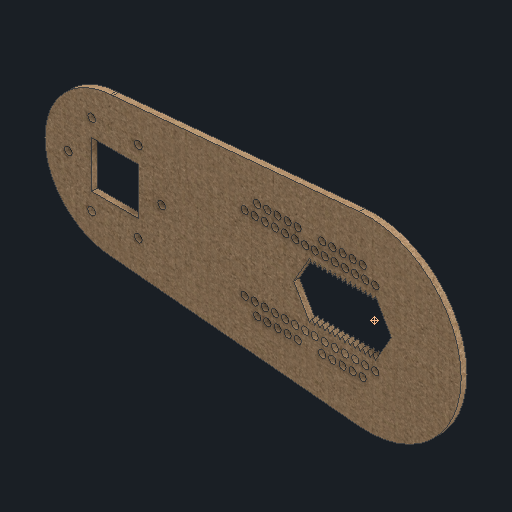
# Autodesk Inventor part: WeightArm
Saved by Autodesk Inventor 2024.1 (Build 281209000, 209)
## iProperties
Created: 2023-10-16
Part Number: WeightArm
Material: MDF Medium Density Fiberboard
Document SubType Name: Modeling
Designer: Brandon
Density: 0.8 g/cm^3
Appearance: Cardboard - Corrugated
Mass: 33.1484 g
Surface Area: 289.834 cm^2
Volume: 41.4355 cm^3
Author: Brandon
Autodesk Inventor part; units mm, degrees
ref_plane "YZ Plane" through (0, 0, 0) normal (1, 0, 0) x (0, 1, 0)
ref_plane "XZ Plane" through (0, 0, 0) normal (0, 1, 0) x (-1, 0, 0)
ref_plane "XY Plane" through (0, 0, 0) normal (0, 0, 1) x (1, 0, 0)
sketch "Sketch1" plane through (0, 0, 0) normal (0, 0, 1) x (1, 0, 0)
  line L0 (-285.1848, -19.0386) -> (264.1554, -38.0771) projected
  arc A0 (264.1554, -38.0771) -> (264.1554, 38.0771) centre (265.475, 0) ccw projected
  line L1 (264.1554, 38.0771) -> (-285.1848, 19.0386) projected
  arc A1 (-285.1848, 19.0386) -> (-285.1848, -19.0386) centre (-284.525, 0) ccw projected
  circle A2 centre (-284.525, -9.525) radius 2 projected
  circle A3 centre (-294.05, 0) radius 2 projected
  circle A4 centre (-284.525, 9.525) radius 2 projected
  circle A5 centre (290.875, 0) radius 2.1 projected
  circle A6 centre (278.175, -21.997) radius 2.1 projected
  circle A7 centre (252.775, -21.997) radius 2.1 projected
  circle A8 centre (278.175, 21.997) radius 2.1 projected
  circle A9 centre (252.775, 21.997) radius 2.1 projected
  line L2 (252.775, -12.7) -> (252.775, 12.7) projected
  line L3 (252.775, 12.7) -> (278.175, 12.7) projected
  line L4 (278.175, 12.7) -> (278.175, -12.7) projected
  line L5 (278.175, -12.7) -> (252.775, -12.7) projected
  circle A10 centre (240.075, 0) radius 2.1 projected
  circle A11 centre (-275, 0) radius 2 projected
  circle A12 centre (265.475, 0) radius 38.1
  line L6 (265.475, 0) -> (402.975, 0)
  arc A13 (398.2829, -50.5828) -> (398.2829, 50.5828) centre (402.975, 0) ccw
  line L7 (261.9559, 37.9371) -> (398.2829, 50.5828)
  line L8 (265.475, 0) -> (375.475, 0)
  line L9 (402.975, 12.7) -> (402.975, -12.7)
  line L10 (404.35, 12.7) -> (401.6, 12.7)
  line L11 (402.975, 12.7) -> (404.35, 15.0816)
  line L12 (402.975, 12.7) -> (405.725, 12.7) construction
  line L13 (404.35, 15.0816) -> (405.725, 12.7)
  line L14 (405.725, 12.7) -> (407.1, 15.0816)
  line L15 (405.725, 12.7) -> (408.475, 12.7) construction
  line L16 (407.1, 15.0816) -> (408.475, 12.7)
  line L17 (402.975, -12.7) -> (404.35, -15.0816)
  line L18 (402.975, -12.7) -> (405.725, -12.7) construction
  line L19 (404.35, -15.0816) -> (405.725, -12.7)
  line L20 (405.725, -12.7) -> (407.1, -15.0816)
  line L21 (405.725, -12.7) -> (408.475, -12.7) construction
  line L22 (407.1, -15.0816) -> (408.475, -12.7)
  line L23 (397.475, 12.7) -> (398.85, 15.0816)
  line L24 (398.85, 15.0816) -> (400.225, 12.7)
  line L25 (397.475, 12.7) -> (400.225, 12.7) construction
  line L26 (400.225, 12.7) -> (401.6, 15.0816)
  line L27 (401.6, 15.0816) -> (402.975, 12.7)
  line L28 (400.225, 12.7) -> (402.975, 12.7) construction
  line L29 (397.475, -12.7) -> (398.85, -15.0816)
  line L30 (397.475, -12.7) -> (400.225, -12.7) construction
  line L31 (400.225, -12.7) -> (401.6, -15.0816)
  line L32 (400.225, -12.7) -> (402.975, -12.7) construction
  line L33 (401.6, -15.0816) -> (402.975, -12.7)
  line L34 (398.85, -15.0816) -> (400.225, -12.7)
  line L35 (391.975, 12.7) -> (393.35, 15.0816)
  line L36 (393.35, 15.0816) -> (394.725, 12.7)
  line L37 (391.975, 12.7) -> (394.725, 12.7) construction
  line L38 (394.725, 12.7) -> (396.1, 15.0816)
  line L39 (396.1, 15.0816) -> (397.475, 12.7)
  line L40 (394.725, 12.7) -> (397.475, 12.7) construction
  line L41 (391.975, -12.7) -> (393.35, -15.0816)
  line L42 (391.975, -12.7) -> (394.725, -12.7) construction
  line L43 (394.725, -12.7) -> (396.1, -15.0816)
  line L44 (394.725, -12.7) -> (397.475, -12.7) construction
  line L45 (396.1, -15.0816) -> (397.475, -12.7)
  line L46 (393.35, -15.0816) -> (394.725, -12.7)
  line L47 (386.475, 12.7) -> (387.85, 15.0816)
  line L48 (387.85, 15.0816) -> (389.225, 12.7)
  line L49 (386.475, 12.7) -> (389.225, 12.7) construction
  line L50 (389.225, 12.7) -> (390.6, 15.0816)
  line L51 (390.6, 15.0816) -> (391.975, 12.7)
  line L52 (389.225, 12.7) -> (391.975, 12.7) construction
  line L53 (386.475, -12.7) -> (387.85, -15.0816)
  line L54 (386.475, -12.7) -> (389.225, -12.7) construction
  line L55 (389.225, -12.7) -> (390.6, -15.0816)
  line L56 (389.225, -12.7) -> (391.975, -12.7) construction
  line L57 (390.6, -15.0816) -> (391.975, -12.7)
  line L58 (387.85, -15.0816) -> (389.225, -12.7)
  line L59 (380.975, 12.7) -> (382.35, 15.0816)
  line L60 (382.35, 15.0816) -> (383.725, 12.7)
  line L61 (380.975, 12.7) -> (383.725, 12.7) construction
  line L62 (383.725, 12.7) -> (385.1, 15.0816)
  line L63 (385.1, 15.0816) -> (386.475, 12.7)
  line L64 (383.725, 12.7) -> (386.475, 12.7) construction
  line L65 (380.975, -12.7) -> (382.35, -15.0816)
  line L66 (380.975, -12.7) -> (383.725, -12.7) construction
  line L67 (383.725, -12.7) -> (385.1, -15.0816)
  line L68 (383.725, -12.7) -> (386.475, -12.7) construction
  line L69 (385.1, -15.0816) -> (386.475, -12.7)
  line L70 (382.35, -15.0816) -> (383.725, -12.7)
  line L71 (375.475, 12.7) -> (376.85, 15.0816)
  line L72 (376.85, 15.0816) -> (378.225, 12.7)
  line L73 (375.475, 12.7) -> (378.225, 12.7) construction
  line L74 (378.225, 12.7) -> (379.6, 15.0816)
  line L75 (379.6, 15.0816) -> (380.975, 12.7)
  line L76 (378.225, 12.7) -> (380.975, 12.7) construction
  line L77 (375.475, -12.7) -> (376.85, -15.0816)
  line L78 (375.475, -12.7) -> (378.225, -12.7) construction
  line L79 (378.225, -12.7) -> (379.6, -15.0816)
  line L80 (378.225, -12.7) -> (380.975, -12.7) construction
  line L81 (379.6, -15.0816) -> (380.975, -12.7)
  line L82 (376.85, -15.0816) -> (378.225, -12.7)
  line L83 (369.975, 12.7) -> (371.35, 15.0816)
  line L84 (371.35, 15.0816) -> (372.725, 12.7)
  line L85 (369.975, 12.7) -> (372.725, 12.7) construction
  line L86 (372.725, 12.7) -> (374.1, 15.0816)
  line L87 (374.1, 15.0816) -> (375.475, 12.7)
  line L88 (372.725, 12.7) -> (375.475, 12.7) construction
  line L89 (369.975, -12.7) -> (371.35, -15.0816)
  line L90 (369.975, -12.7) -> (372.725, -12.7) construction
  line L91 (372.725, -12.7) -> (374.1, -15.0816)
  line L92 (372.725, -12.7) -> (375.475, -12.7) construction
  line L93 (374.1, -15.0816) -> (375.475, -12.7)
  line L94 (371.35, -15.0816) -> (372.725, -12.7)
  line L95 (408.475, 12.7) -> (415.8073, 0)
  line L96 (415.8073, 0) -> (408.475, -12.7)
  line L97 (369.975, -12.7) -> (362.6427, 0)
  line L98 (369.975, 12.7) -> (362.6427, 0)
  line L99 (261.9559, -37.9371) -> (398.2829, -50.5828)
  line L100 (-195.625, 1.5875) -> (-195.625, -1.5875) projected
  line L101 (-195.625, -1.5875) -> (-221.025, -1.5875) projected
  line L102 (-221.025, -1.5875) -> (-221.025, 1.5875) projected
  line L103 (-221.025, 1.5875) -> (-195.625, 1.5875) projected
  line L104 (-170.225, -1.5875) -> (-170.225, 1.5875) projected
  line L105 (-170.225, 1.5875) -> (-144.825, 1.5875) projected
  line L106 (-144.825, 1.5875) -> (-144.825, -1.5875) projected
  line L107 (-144.825, -1.5875) -> (-170.225, -1.5875) projected
  line L108 (-119.425, -1.5875) -> (-119.425, 1.5875) projected
  line L109 (-119.425, 1.5875) -> (-94.025, 1.5875) projected
  line L110 (-94.025, 1.5875) -> (-94.025, -1.5875) projected
  line L111 (-94.025, -1.5875) -> (-119.425, -1.5875) projected
  line L112 (-68.625, -1.5875) -> (-68.625, 1.5875) projected
  line L113 (-68.625, 1.5875) -> (-43.225, 1.5875) projected
  line L114 (-43.225, 1.5875) -> (-43.225, -1.5875) projected
  line L115 (-43.225, -1.5875) -> (-68.625, -1.5875) projected
  line L116 (-17.825, -1.5875) -> (-17.825, 1.5875) projected
  line L117 (-17.825, 1.5875) -> (7.575, 1.5875) projected
  line L118 (7.575, 1.5875) -> (7.575, -1.5875) projected
  line L119 (7.575, -1.5875) -> (-17.825, -1.5875) projected
  line L120 (32.975, -1.5875) -> (32.975, 1.5875) projected
  line L121 (32.975, 1.5875) -> (58.375, 1.5875) projected
  line L122 (58.375, 1.5875) -> (58.375, -1.5875) projected
  line L123 (58.375, -1.5875) -> (32.975, -1.5875) projected
  line L124 (83.775, -1.5875) -> (83.775, 1.5875) projected
  line L125 (83.775, 1.5875) -> (109.175, 1.5875) projected
  line L126 (109.175, 1.5875) -> (109.175, -1.5875) projected
  line L127 (109.175, -1.5875) -> (83.775, -1.5875) projected
  line L128 (134.575, -1.5875) -> (134.575, 1.5875) projected
  line L129 (134.575, 1.5875) -> (159.975, 1.5875) projected
  line L130 (159.975, 1.5875) -> (159.975, -1.5875) projected
  line L131 (159.975, -1.5875) -> (134.575, -1.5875) projected
  line L132 (185.375, -1.5875) -> (185.375, 1.5875) projected
  line L133 (185.375, 1.5875) -> (210.775, 1.5875) projected
  line L134 (210.775, 1.5875) -> (210.775, -1.5875) projected
  line L135 (210.775, -1.5875) -> (185.375, -1.5875) projected
  point P0 (0, 0)
  point P1 (265.475, 38.1)
  point P2 (264.1554, 38.0771)
  point P3 (263.0536, -38.039)
  point P4 (263.0536, 38.039)
  dimension "d0" = 137.5
  dimension "d1" = 101.6
  dimension "d2" = 110
  dimension "d3" = 25.4
  dimension "d4" = 2.75
  dimension "d5" = 60
  dimension "d6" = 2.75
  dimension "d7" = 60
  dimension "d8" = 2.75
  dimension "d11" = 5.5
  constraints: 188 end point, 5 horizontal, 4 point on circle, 4 symmetric about line, 4 tangent, 3 equal length, 2 centre point, 2 coincident, 2 collinear, 2 midpoint, 2 point on line, 1 concentric, 1 vertical, 132 other
  measures "d0" distance of L6.end L6.start
  measures "d1" diameter of A13
  measures "d2" distance of L6.start L8.end
  measures "d3" distance of L9.start L9.end
  measures "d4" distance of L10.start L10.end
  measures "d5" angle of L12 L11
  measures "d6" distance of L9.start L12.end
  measures "d7" angle of L15 L14
  measures "d8" distance of L12.end L15.end
  measures "d11" distance of L11.end L23.end
extrude "Extrusion1" add sketch "Sketch1" along normal blind 3.175 contours L0 A0 L1 L7 A13 L99 | A12 A0
sketch "Sketch2" plane through (0, 0, 0) normal (0, 0, -1) x (-1, 0, 0)
  line L0 (-375.5993, 0) -> (-368.3167, 0)
  circle A0 centre (-407.1, 20.1616) radius 2
  circle A1 centre (-400.225, 26.5116) radius 2
  circle A2 centre (-401.6, 20.1616) radius 2
  circle A3 centre (-394.725, 26.5116) radius 2
  circle A4 centre (-396.1, 20.1616) radius 2
  circle A5 centre (-390.6, 20.1616) radius 2
  circle A6 centre (-389.225, 26.5116) radius 2
  circle A7 centre (-385.1, 20.1616) radius 2
  circle A8 centre (-383.725, 26.5116) radius 2
  circle A9 centre (-378.225, 26.5116) radius 2
  circle A10 centre (-379.6, 20.1616) radius 2
  circle A11 centre (-374.1, 20.1616) radius 2
  circle A12 centre (-369, 20.1616) radius 2
  circle A13 centre (-364.875, 26.5116) radius 2
  circle A14 centre (-363.5, 20.1616) radius 2
  circle A15 centre (-359.375, 26.5116) radius 2
  circle A16 centre (-358, 20.1616) radius 2
  circle A17 centre (-353.875, 26.5116) radius 2
  circle A18 centre (-352.5, 20.1616) radius 2
  circle A19 centre (-348.375, 26.5116) radius 2
  circle A20 centre (-347, 20.1616) radius 2
  circle A21 centre (-342.875, 26.5116) radius 2
  circle A22 centre (-341.5, 20.1616) radius 2
  circle A23 centre (-336, 20.1616) radius 2
  circle A24 centre (-407.1, -20.1616) radius 2
  circle A25 centre (-400.225, -26.5116) radius 2
  circle A26 centre (-401.6, -20.1616) radius 2
  circle A27 centre (-394.725, -26.5116) radius 2
  circle A28 centre (-396.1, -20.1616) radius 2
  circle A29 centre (-390.6, -20.1616) radius 2
  circle A30 centre (-389.225, -26.5116) radius 2
  circle A31 centre (-385.1, -20.1616) radius 2
  circle A32 centre (-383.725, -26.5116) radius 2
  circle A33 centre (-378.225, -26.5116) radius 2
  circle A34 centre (-379.6, -20.1616) radius 2
  circle A35 centre (-374.1, -20.1616) radius 2
  circle A36 centre (-369, -20.1616) radius 2
  circle A37 centre (-364.875, -26.5116) radius 2
  circle A38 centre (-363.5, -20.1616) radius 2
  circle A39 centre (-359.375, -26.5116) radius 2
  circle A40 centre (-358, -20.1616) radius 2
  circle A41 centre (-353.875, -26.5116) radius 2
  circle A42 centre (-352.5, -20.1616) radius 2
  circle A43 centre (-348.375, -26.5116) radius 2
  circle A44 centre (-347, -20.1616) radius 2
  circle A45 centre (-342.875, -26.5116) radius 2
  circle A46 centre (-341.5, -20.1616) radius 2
  circle A47 centre (-336, -20.1616) radius 2
  point P0 (0, 0)
  point P1 (-402.975, 26.5116)
  point P2 (-398.85, 20.1616)
  point P3 (-360.75, 20.1616)
  point P4 (-407.1, -20.1616)
  point P5 (-402.975, -26.5116)
  point P6 (-398.85, -20.1616)
  point P7 (-369, -20.1616)
  point P8 (-364.875, -26.5116)
  point P9 (-360.75, -20.1616)
  point P10 (-407.1, 15.0816)
  point P11 (-404.35, 15.0816)
  point P12 (-404.35, 20.1616)
  point P13 (-396.1, 20.1616)
  point P14 (-366.25, 20.1616)
  point P15 (-362.125, 26.5116)
  point P16 (-358, 20.1616)
  point P17 (-404.35, -20.1616)
  point P18 (-400.225, -26.5116)
  point P19 (-396.1, -20.1616)
  point P20 (-366.25, -20.1616)
  point P21 (-362.125, -26.5116)
  point P22 (-358, -20.1616)
  point P23 (-397.475, 26.5116)
  point P24 (-393.35, 20.1616)
  point P25 (-355.25, 20.1616)
  point P26 (-401.6, -20.1616)
  point P27 (-397.475, -26.5116)
  point P28 (-393.35, -20.1616)
  point P29 (-363.5, -20.1616)
  point P30 (-359.375, -26.5116)
  point P31 (-355.25, -20.1616)
  point P32 (-398.85, 20.1616)
  point P33 (-390.6, 20.1616)
  point P34 (-360.75, 20.1616)
  point P35 (-356.625, 26.5116)
  point P36 (-352.5, 20.1616)
  point P37 (-398.85, -20.1616)
  point P38 (-394.725, -26.5116)
  point P39 (-390.6, -20.1616)
  point P40 (-360.75, -20.1616)
  point P41 (-356.625, -26.5116)
  point P42 (-352.5, -20.1616)
  point P43 (-391.975, 26.5116)
  point P44 (-387.85, 20.1616)
  point P45 (-349.75, 20.1616)
  point P46 (-396.1, -20.1616)
  point P47 (-391.975, -26.5116)
  point P48 (-387.85, -20.1616)
  point P49 (-358, -20.1616)
  point P50 (-353.875, -26.5116)
  point P51 (-349.75, -20.1616)
  point P52 (-393.35, 20.1616)
  point P53 (-385.1, 20.1616)
  point P54 (-355.25, 20.1616)
  point P55 (-351.125, 26.5116)
  point P56 (-347, 20.1616)
  point P57 (-393.35, -20.1616)
  point P58 (-389.225, -26.5116)
  point P59 (-385.1, -20.1616)
  point P60 (-355.25, -20.1616)
  point P61 (-351.125, -26.5116)
  point P62 (-347, -20.1616)
  point P63 (-386.475, 26.5116)
  point P64 (-382.35, 20.1616)
  point P65 (-344.25, 20.1616)
  point P66 (-390.6, -20.1616)
  point P67 (-386.475, -26.5116)
  point P68 (-382.35, -20.1616)
  point P69 (-352.5, -20.1616)
  point P70 (-348.375, -26.5116)
  point P71 (-344.25, -20.1616)
  point P72 (-387.85, 20.1616)
  point P73 (-349.75, 20.1616)
  point P74 (-345.625, 26.5116)
  point P75 (-387.85, -20.1616)
  point P76 (-383.725, -26.5116)
  point P77 (-379.6, -20.1616)
  point P78 (-349.75, -20.1616)
  point P79 (-345.625, -26.5116)
  point P80 (-341.5, -20.1616)
  point P81 (-380.975, 26.5116)
  point P82 (-376.85, 20.1616)
  point P83 (-338.75, 20.1616)
  point P84 (-385.1, -20.1616)
  point P85 (-380.975, -26.5116)
  point P86 (-376.85, -20.1616)
  point P87 (-347, -20.1616)
  point P88 (-342.875, -26.5116)
  point P89 (-338.75, -20.1616)
  point P90 (-382.35, 20.1616)
  point P91 (-344.25, 20.1616)
  point P92 (-340.125, 26.5116)
  point P93 (-382.35, -20.1616)
  point P94 (-378.225, -26.5116)
  point P95 (-374.1, -20.1616)
  point P96 (-344.25, -20.1616)
  point P97 (-340.125, -26.5116)
  point P98 (-336, -20.1616)
  point P99 (-402.975, -26.5116)
  point P100 (-398.85, -20.1616)
  point P101 (-360.75, -20.1616)
  point P102 (-404.35, -20.1616)
  point P103 (-396.1, -20.1616)
  point P104 (-366.25, -20.1616)
  point P105 (-362.125, -26.5116)
  point P106 (-358, -20.1616)
  point P107 (-397.475, -26.5116)
  point P108 (-393.35, -20.1616)
  point P109 (-355.25, -20.1616)
  point P110 (-398.85, -20.1616)
  point P111 (-390.6, -20.1616)
  point P112 (-360.75, -20.1616)
  point P113 (-356.625, -26.5116)
  point P114 (-352.5, -20.1616)
  point P115 (-391.975, -26.5116)
  point P116 (-387.85, -20.1616)
  point P117 (-349.75, -20.1616)
  point P118 (-393.35, -20.1616)
  point P119 (-385.1, -20.1616)
  point P120 (-355.25, -20.1616)
  point P121 (-351.125, -26.5116)
  point P122 (-347, -20.1616)
  point P123 (-386.475, -26.5116)
  point P124 (-382.35, -20.1616)
  point P125 (-344.25, -20.1616)
  point P126 (-387.85, -20.1616)
  point P127 (-349.75, -20.1616)
  point P128 (-345.625, -26.5116)
  point P129 (-380.975, -26.5116)
  point P130 (-376.85, -20.1616)
  point P131 (-338.75, -20.1616)
  point P132 (-382.35, -20.1616)
  point P133 (-344.25, -20.1616)
  point P134 (-340.125, -26.5116)
  dimension "d20" = 2.75
  dimension "d25" = 4
  dimension "d26" = 4
  dimension "d27" = 4
  dimension "d28" = 4
  dimension "d29" = 4
  dimension "d30" = 4
  dimension "d31" = 4
  dimension "d32" = 4
  dimension "d33" = 4
  dimension "d34" = 4
  dimension "d35" = 4
  dimension "d36" = 4
  dimension "d37" = 4
  dimension "d38" = 4
  dimension "d39" = 4
  dimension "d40" = 4
  dimension "d41" = 4
  dimension "d42" = 4
  dimension "d43" = 4
  dimension "d44" = 4
  dimension "d45" = 4
  dimension "d46" = 4
  dimension "d47" = 4
  dimension "d48" = 4
  constraints: 84 symmetric about line, 48 centre point, 48 coincident, 3 horizontal, 2 end point, 134 other
  measures "d20" distance of point (-402.975, 26.512) point (-400.225, 26.512)
  measures "d25" diameter of A0
  measures "d26" diameter of A1
  measures "d27" diameter of A2
  measures "d28" diameter of A3
  measures "d29" diameter of A4
  measures "d30" diameter of A5
  measures "d31" diameter of A6
  measures "d32" diameter of A7
  measures "d33" diameter of A8
  measures "d34" diameter of A9
  measures "d35" diameter of A10
  measures "d36" diameter of A11
  measures "d37" diameter of A12
  measures "d38" diameter of A13
  measures "d39" diameter of A14
  measures "d40" diameter of A15
  measures "d41" diameter of A16
  measures "d42" diameter of A17
  measures "d43" diameter of A18
  measures "d44" diameter of A19
  measures "d45" diameter of A20
  measures "d46" diameter of A21
  measures "d47" diameter of A22
  measures "d48" diameter of A23
extrude "Extrusion2" cut sketch "Sketch2" against normal through all
body "Solid1"
